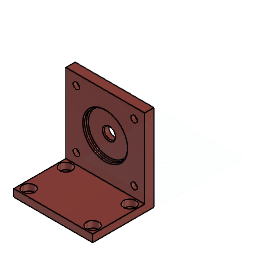
SoporteP v5 (Autodesk Fusion 360 design; units mm, degrees)
Autodesk Fusion 360 part; units mm, degrees
sketch "Sketch1" plane through (0, 0, 0) normal (0, 0, 1) x (1, 0, 0)
  line L0 (21.125, 21.125) -> (-21.125, 21.125)
  line L1 (-21.125, 21.125) -> (-21.125, -21.125)
  line L2 (-21.125, -21.125) -> (21.125, -21.125)
  line L3 (21.125, -21.125) -> (21.125, 21.125)
  line L4 (21.125, 21.125) -> (-21.125, -21.125) construction
  line L5 (-21.125, 21.125) -> (21.125, -21.125) construction
  dimension "d1" = 42.25
  dimension "d2" = 42.25
  constraint horizontal L0
  constraint perpendicular L0 L1
  constraint parallel L0 L2
  constraint parallel L1 L3
  constraint coincident L4 origin
  constraint coincident L5 origin
  measures "d1" distance of L1.end L2.end
  measures "d2" distance of L0.end L1.end
extrude "Extrude1" add sketch "Sketch1" along normal blind 5
sketch "Sketch2" plane through (0, 0, 5) normal (0, 0, 1) x (-1, 0, 0)
  line L0 (-21.125, 21.125) -> (-21.125, -21.125)
  line L1 (-21.125, -21.125) -> (21.125, -21.125)
  line L2 (21.125, -21.125) -> (21.125, 21.125)
  line L3 (21.125, 21.125) -> (-21.125, 21.125)
  circle A0 centre (0, 0) radius 11.5
  line L4 (-21.125, 0) -> (21.125, 0) construction
  line L5 (0, -21.125) -> (0, 21.125) construction
  point P0 (-15.5, -15.5)
  point P1 (15.5, -15.5)
  point P2 (-15.5, 15.5)
  point P3 (15.5, 15.5)
  dimension "d5" = 23
  dimension "d32" = 5.625
  dimension "d33" = 5.625
  constraint coincident A0.centre origin
  constraint midpoint L0 L4.start
  constraint midpoint L2 L4.end
  constraint midpoint L1 L5.start
  constraint midpoint L3 L5.end
  constraint symmetric P0 L5 P1
  constraint symmetric P0 L4 P2
  constraint symmetric L4 P1 P3
  measures "d5" diameter of A0
  measures "d32" distance of L0 P0
  measures "d33" distance of L1 P0
extrude "Extrude2" cut sketch "Sketch2" against normal blind 2 contours A0
sketch "Sketch3" plane through (0, 0, 3) normal (0, 0, 1) x (-1, 0, 0)
  circle A0 centre (0, 0) radius 11.5
  circle A1 centre (0, 0) radius 3
  dimension "d8" = 6
  constraint coincident A0.centre A1.centre
  measures "d8" diameter of A1
extrude "Extrude3" cut sketch "Sketch3" against normal blind 3 contours A1
sketch "Sketch6" plane through (0, 0, 0) normal (0, 0, -1) x (1, 0, 0)
  circle A0 centre (0, 0) radius 3
  line L0 (21.125, -21.125) -> (21.125, 21.125)
  line L1 (21.125, 21.125) -> (-21.125, 21.125)
  line L2 (-21.125, 21.125) -> (-21.125, -21.125)
  line L3 (-21.125, -21.125) -> (21.125, -21.125)
extrude "Extrude4" add 1 faces at (-7.0417, -21.125, 1.6667) along direction (0, -1, 0) blind 5
sketch "Sketch5" plane through (0, 0, 5) normal (0, 0, 1) x (-1, 0, 0)
  circle A0 centre (0, 0) radius 11.5
  line L0 (-21.125, 26.125) -> (-21.125, -21.125)
  line L1 (-21.125, -21.125) -> (21.125, -21.125)
  line L2 (21.125, -21.125) -> (21.125, 26.125)
  line L3 (21.125, 26.125) -> (-21.125, 26.125)
  line L4 (21.125, 23.625) -> (-21.125, 23.625)
  line L5 (21.125, -21.125) -> (-21.125, -21.125)
  line L6 (-21.125, -21.125) -> (-21.125, 21.125)
  dimension "d15" = 2.5
  constraint coincident L2 L4.start
  constraint coincident L0 L4.end
  constraint perpendicular L0 L4
  measures "d15" distance of L3 L4
extrude "Extrude5" add sketch "Sketch5" along normal blind 34 contours L0 L2 L3 L4
fillet "Fillet1" radius 0.5 2 faces at (-8.6127, 0.7204, 3) (-11.4857, 0.5732, 3.6667)
sketch "Sketch11" plane through (0, 0, 0) normal (0, 0, -1) x (1, 0, 0)
  line L0 (0, -0.125) -> (0, -42.125) construction
  line L1 (21.1283, 0) -> (-21.125, 0) construction
  line L2 (21.125, -21.125) -> (21.125, 21.125)
  line L3 (-21.125, -21.125) -> (21.125, -21.125)
  line L4 (-21.125, 21.125) -> (-21.125, -21.125)
  point P0 (15.5, -15.5)
  point P1 (-15.5, -15.5)
  point P2 (15.5, 15.5)
  point P3 (-15.5, 15.5)
  dimension "d36" = 5.625
  dimension "d37" = 5.625
  constraint vertical L0
  constraint perpendicular L0 L1
  constraint symmetric L0 P0 P1
  constraint midpoint L0 L3
  constraint symmetric L1 P0 P2
  constraint symmetric L1 P1 P3
  constraint midpoint L1.end L4
  measures "d36" distance of P0 L2
  measures "d37" distance of P0 L3
hole "Hole2" at (15.5, 15.5, 0) at (-15.5, 15.5, 0) at (-15.5, -15.5, 0) at (15.5, -15.5, 0) direction (0, 0, 1) diameter 3.4 depth 5 tip angle 118 counterbore diameter 6.5 counterbore depth 3
move_body "Move1" bodies 1 to x (1, 0, 0) y (0, 0, 1) z (0, -1, 0) at (0, -26.125, 26.125)
extrude "Extrude6" cut 1 faces at (7.0417, -65.125, 1.6667) along direction (0, 1, 0) blind 6.139
extrude "Extrude7" add 1 faces at (-7.0417, -40.412, 2.5) along direction (0, 0, 1) blind 2
extrude "Extrude8" cut 1 faces at (-7.0417, -37.0787, 0) along direction (0, 0, 1) blind 2.5
sketch "Sketch14" plane through (0, 0, 4.5) normal (0, 0, 1) x (-1, 0, 0)
  line L0 (21.125, 58.986) -> (-21.125, 58.986)
  line L1 (-21.125, 58.986) -> (-21.125, 31.125)
  line L2 (-21.125, 31.125) -> (21.125, 31.125)
  line L3 (21.125, 31.125) -> (21.125, 58.986)
  line L4 (-21.125, 45.0555) -> (21.125, 45.0555) construction
  line L5 (0, 58.986) -> (0, 31.125) construction
  point P0 (-17.125, 35.125)
  point P1 (-17.125, 54.986)
  point P2 (17.125, 35.125)
  point P3 (17.125, 54.986)
  dimension "d59" = 4
  dimension "d60" = 4
  constraint midpoint L1 L4.start
  constraint midpoint L3 L4.end
  constraint midpoint L0 L5.start
  constraint midpoint L2 L5.end
  constraint symmetric L4 P0 P1
  constraint symmetric L5 P0 P2
  constraint symmetric L5 P1 P3
  measures "d59" distance of L1 P0
  measures "d60" distance of L2 P0
extrude "Extrude11" add 1 faces at (-7.0417, -37.0787, 2.5) along direction (0, 0, -1) blind 1.5
hole "Hole3" at (-17.125, -35.125, 4.5) at (-17.125, -54.986, 4.5) at (17.125, -54.986, 4.5) at (17.125, -35.125, 4.5) direction (0, 0, -1) diameter 3.4 depth 7 tip angle 180 counterbore diameter 6.5 counterbore depth 3
extrude "Extrude12" add 1 faces at (-4.7701, -42.287, 4.5) along direction (0, 0, 1) blind 0.5
